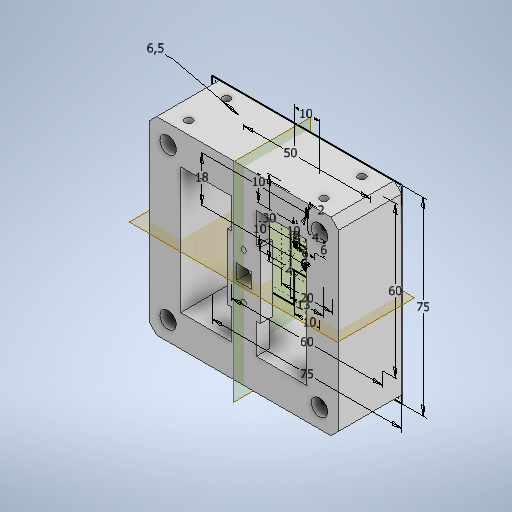
# Autodesk Inventor part: camera_60mm
Saved by Autodesk Inventor 2025.1 (Build 291241000, 241)
## iProperties
Created: 2024-11-22
Part Number: camera_60mm
Material: Ogólny
Document SubType Name: Modeling
Designer: PC
Density: 1 g/cm^3
Appearance: Domyślna
Author: PC
Autodesk Inventor part; units mm, degrees
ref_plane "YZ Plane" through (0, 0, 0) normal (1, 0, 0) x (0, 1, 0)
ref_plane "XZ Plane" through (0, 0, 0) normal (0, 1, 0) x (-1, 0, 0)
ref_plane "XY Plane" through (0, 0, 0) normal (0, 0, 1) x (1, 0, 0)
sketch "Szkic1" plane through (0, 0, 0) normal (0, 0, 1) x (1, 0, 0)
  line L0 (-24.2993, 7.2735) -> (25.7007, 7.2735) construction
  circle A0 centre (60, 60) radius 3.25
  circle A1 centre (0, 60) radius 3.25
  line L1 (40, 45) -> (20, 45) construction
  line L2 (20, 45) -> (20, 15) construction
  line L3 (20, 15) -> (40, 15) construction
  line L4 (40, 15) -> (40, 45) construction
  line L5 (40, 45) -> (20, 15) construction
  line L6 (20, 45) -> (40, 15) construction
  line L7 (30, 45) -> (30, 15) construction
  circle A2 centre (30, 39) radius 1
  circle A3 centre (30, 21) radius 1
  circle A4 centre (30, 39) radius 2
  circle A5 centre (30, 21) radius 2
  line L8 (23.5, 17) -> (36.5, 17)
  line L9 (33, 33) -> (27, 33)
  line L10 (27, 33) -> (27, 27)
  line L11 (27, 27) -> (33, 27)
  line L12 (33, 27) -> (33, 33)
  line L13 (33, 33) -> (27, 27) construction
  line L14 (27, 33) -> (33, 27) construction
  line L15 (30, 39) -> (30, 21) construction
  line L16 (0, 60) -> (60, 60) construction
  line L17 (60, 60) -> (60, 0) construction
  line L18 (60, 0) -> (0, 0) construction
  line L19 (0, 0) -> (0, 60) construction
  circle A6 centre (0, 0) radius 3.25
  circle A7 centre (60, 0) radius 3.25
  line L20 (23.5, 43) -> (36.5, 43)
  line L21 (-7.5, 67.5) -> (67.5, 67.5)
  line L22 (67.5, 67.5) -> (67.5, -7.5)
  line L23 (67.5, -7.5) -> (-7.5, -7.5)
  line L24 (-7.5, -7.5) -> (-7.5, 67.5)
  line L25 (-7.5, 67.5) -> (67.5, -7.5) construction
  line L26 (67.5, 67.5) -> (-7.5, -7.5) construction
  line L27 (23.5, 17) -> (23.5, 25)
  line L28 (23.5, 35) -> (23.5, 43)
  line L29 (36.5, 43) -> (36.5, 35)
  line L30 (36.5, 25) -> (36.5, 17)
  line L31 (5, 5) -> (5, 30.7649)
  line L32 (5, 40.7649) -> (5, 55)
  line L33 (55, 55) -> (55, 40.7649)
  line L34 (55, 30.7649) -> (55, 5)
  line L35 (5, 55) -> (5, 5) construction
  line L36 (55, 5) -> (55, 55) construction
  line L37 (23.5, 35) -> (23.5, 25)
  line L38 (36.5, 25) -> (36.5, 35)
  line L39 (25, 35) -> (35, 35)
  line L40 (35, 35) -> (35, 25)
  line L41 (35, 25) -> (25, 25)
  line L42 (25, 25) -> (25, 35)
  line L43 (25.5, 34.5) -> (34.5, 34.5)
  line L44 (34.5, 34.5) -> (34.5, 25.5)
  line L45 (34.5, 25.5) -> (25.5, 25.5)
  line L46 (25.5, 25.5) -> (25.5, 34.5)
  line L47 (25, 55) -> (25, 43)
  line L48 (25, 17) -> (25, 5)
  line L49 (35, 55) -> (35, 43)
  line L50 (35, 17) -> (35, 5)
  line L51 (5, 40.7649) -> (5, 30.7649)
  line L52 (55, 40.7649) -> (55, 30.7649)
  line L53 (55, 5) -> (35, 5)
  line L54 (25, 5) -> (5, 5)
  line L55 (5, 55) -> (25, 55)
  line L56 (35, 55) -> (55, 55)
  line L57 (25, 55) -> (35, 55) construction
  line L58 (25, 5) -> (35, 5) construction
  point P0 (30, 30)
  point P1 (37.6222, 60)
  point P2 (33, 30)
  point P3 (60, 30)
  point P4 (30, 27)
  point P5 (30, 0)
  point P6 (30, 30)
  point P7 (5, 30)
  point P8 (-7.5, 30)
  point P9 (30, 5)
  point P10 (30, -7.5)
  point P11 (30, 43)
  point P12 (30, 25.5)
  point P13 (30, 25)
  point P14 (30, 55)
  dimension "d3" = 20
  dimension "d4" = 30
  dimension "d5" = 2
  dimension "d6" = 18
  dimension "d7" = 4
  dimension "d8" = 4
  dimension "d9" = 6
  dimension "d10" = 6
  dimension "d11" = 13
  dimension "d14" = 60
  dimension "d15" = 60
  dimension "d16" = 6.5
  dimension "d19" = 75
  dimension "d20" = 75
  dimension "d21" = 50
  dimension "d22" = 10
  dimension "d23" = 10
  dimension "d41" = 10
  dimension "d42" = 9
  dimension "d54" = 10
  dimension "d55" = 10
  constraints: 116 end point, 22 parallel, 21 perpendicular, 19 midpoint, 11 point on line, 10 collinear, 9 horizontal, 8 centre point, 6 coincident, 6 vertical alignment, 4 equal radius, 4 horizontal alignment, 2 vertical, 10 other
  measures "d3" distance of L3.end L2.end
  measures "d4" distance of L2.end L1.end
  measures "d5" diameter of A2
  measures "d6" distance of A3.centre A2.centre
  measures "d7" diameter of A4
  measures "d8" diameter of A5
  measures "d9" distance of L11.end L9.start
  measures "d10" distance of L10.end L11.end
  measures "d11" distance of L8.start L8.end
  measures "d14" distance of L17.end L18.end
  measures "d15" distance of L16.end L17.end
  measures "d16" diameter of A1
  measures "d19" distance of L22.end L23.end
  measures "d20" distance of L21.end L22.end
  measures "d21" distance of L32.end L33.start
  measures "d22" distance between parallel lines of L9 L20
  measures "d23" distance between parallel lines of L8 L11
  measures "d41" distance of L41.end L39.start
  measures "d42" distance of L45.end L43.start
  measures "d54" distance between parallel lines of L49 L47
  measures "d55" distance between parallel lines of L50 L48
extrude "Wyciągnięcie proste1" add sketch "Szkic1" along normal blind 25 contours A4 | A5 | L27 L37 L28 L20 L29 L38 L30 L8 | L21 L22 L23 L24 | L39 L40 L41 L42 | L43 L44 L45 L46
sketch "Szkic5" plane through (0, 0, 0) normal (0, 0, -1) x (-1, 0, 0)
  line L0 (-55, 25) -> (-55, 5) projected
  line L1 (-5, 55) -> (-55, 55) projected
  line L2 (-55, 5) -> (-5, 5)
  line L3 (-5, 5) -> (-5, 55)
  line L4 (-5, 55) -> (-55, 55)
  line L5 (-55, 55) -> (-55, 5)
  point P0 (0, 0)
  point P1 (-55, 55)
  constraints: 8 end point, 2 parallel, 1 horizontal, 1 perpendicular
extrude "Wyciągnięcie proste7" cut sketch "Szkic5" against normal blind 20
extrude "Wyciągnięcie proste2" add sketch "Szkic1" against normal blind 8 from surface at 25 contours A4 | A5
chamfer "Faza2" distance 3 angle 45 4 edges at (67.5, 67.5, 12.5) (-7.5, 67.5, 12.5) (-7.5, -7.5, 12.5) (67.5, -7.5, 12.5)
sketch "Szkic3" plane through (-4.5, 67.5, 0) normal (0, 1, 0) x (1, 0, 0)
  line L0 (7.75, -25) -> (7.75, 0) construction
  line L1 (1.25, -25) -> (1.25, 0) construction
  circle A0 centre (7.75, -5) radius 1.5
  circle A1 centre (7.75, -20) radius 1.5
  line L2 (69, 0) -> (0, 0) projected
  line L3 (69, -25) -> (0, -25) projected
  point P0 (4.5, 0)
  dimension "d46" = 3
  dimension "d47" = 3
  dimension "d48" = 5
  dimension "d49" = 5
  constraints: 2 centre point, 2 point on line
  measures "d46" diameter of A0
  measures "d47" diameter of A1
  measures "d48" distance from line of L2 A0.centre
  measures "d49" distance from line of L3 A1.centre
extrude "Wyciągnięcie proste6" cut sketch "Szkic3" against normal blind 10.5
ref_plane "Płaszczyzna konstrukcyjna1" through (30, -4.5, 0) normal (-1, 0, 0) x (0, 0, 1)
ref_plane "Płaszczyzna konstrukcyjna2" through (-4.5, 30, 0) normal (0, 1, 0) x (1, 0, 0)
mirror "Odbij1" about plane through (30, -4.5, 0) normal (-1, 0, 0) of "Wyciągnięcie proste6"
mirror "Odbij2" about plane through (30, -4.5, 0) normal (-1, 0, 0) of "Wyciągnięcie proste6", "Odbij1"
mirror "Odbij3" about plane through (-4.5, 30, 0) normal (0, 1, 0) of "Wyciągnięcie proste6", "Odbij1"
